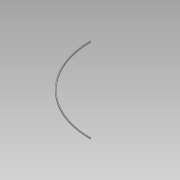
# Autodesk Inventor part: test_ring
Saved by Autodesk Inventor 2019.3 (Build 233278000, 278)
## iProperties
Created: 2019-03-02
Part Number: test_ring
Material: Generic
Document SubType Name: Modeling
Designer: WW
Density: 1 g/cm^3
Appearance: Default
Author: WW
Autodesk Inventor part; units mm, degrees
ref_plane "YZ Plane" through (0, 0, 0) normal (1, 0, 0) x (0, 1, 0)
ref_plane "XZ Plane" through (0, 0, 0) normal (0, 1, 0) x (-1, 0, 0)
ref_plane "XY Plane" through (0, 0, 0) normal (0, 0, 1) x (1, 0, 0)
sketch "Sketch1" plane through (0, 0, 0) normal (0, 1, 0) x (-1, 0, 0)
  circle A0 centre (0, 0) radius 118
  circle A1 centre (0, 0) radius 119
  dimension "d0" = 236
  dimension "d1" = 1
  constraints: 2 centre point, 1 coincident
  measures "d0" diameter of A0
  measures "d1" radial gap between concentric circles of A0 A1
extrude "Extrusion1" add sketch "Sketch1" along normal blind 1
sketch "Sketch2" plane through (0, 1, 0) normal (0, 1, 0) x (1, 0, 0)
  circle A0 centre (0, 0) radius 119 construction
  line L0 (0, -119) -> (-119, -119)
  line L1 (-119, -119) -> (-119, 0)
  line L2 (-119, 0) -> (0, 0)
  line L3 (0, 0) -> (0, -119)
  line L4 (-119, -119) -> (127.2193, -119)
  line L5 (127.2193, -119) -> (127.2193, 155.2075)
  line L6 (127.2193, 155.2075) -> (-119, 155.2075)
  line L7 (-119, 155.2075) -> (-119, -119)
  constraints: 16 end point, 4 parallel, 2 horizontal, 2 perpendicular, 2 point on circle
extrude "Extrusion2" cut sketch "Sketch2" along normal through all both and the other way through all contours L3 L2 L7 L6 L5 L4
body "Solid1"
